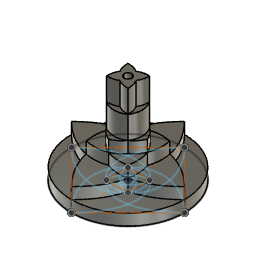
mandala v8 (Autodesk Fusion 360 design; units mm, degrees)
Autodesk Fusion 360 part; units mm, degrees
sketch "Sketch1" plane through (0, 0, 0) normal (0, 0, 1) x (1, 0, 0)
  circle A0 centre (0, 0) radius 25
  line L0 (-25, 0) -> (0, 25)
  line L1 (0, 25) -> (25, 0)
  line L2 (25, 0) -> (0, -25)
  line L3 (0, -25) -> (-25, 0)
  spline S0 degree 4 poles (-25, 0) (0, 25) (25, 0) (0, -25) (-25, 0) knots 0 0 0 0 0 1 1 1 1 1
  line L4 (0, 25) -> (0, -25) construction
  spline S1 degree 4 poles (25, 0) (0, 25) (-25, 0) (0, -25) (25, 0) knots 0 0 0 0 0 1 1 1 1 1
  line L5 (25, 0) -> (0, 25)
  line L6 (0, 25) -> (-25, 0)
  line L7 (-25, 0) -> (0, -25)
  line L8 (0, -25) -> (25, 0)
  line L9 (0, 25) -> (-25, 0)
  line L10 (-25, 0) -> (0, -25)
  line L11 (0, -25) -> (25, 0)
  line L12 (25, 0) -> (0, 25)
  spline S2 degree 4 poles (0, 25) (-25, 0) (0, -25) (25, 0) (0, 25) knots 0 0 0 0 0 1 1 1 1 1
  line L13 (0, -25) -> (25, 0)
  line L14 (25, 0) -> (0, 25)
  line L15 (0, 25) -> (-25, 0)
  line L16 (-25, 0) -> (0, -25)
  spline S3 degree 4 poles (0, -25) (25, 0) (0, 25) (-25, 0) (0, -25) knots 0 0 0 0 0 1 1 1 1 1
  line L17 (-4.7761, 4.7761) -> (4.7922, 4.7652)
  line L18 (4.7922, 4.7652) -> (4.7741, -4.7761)
  line L19 (4.7741, -4.7761) -> (-4.7761, -4.7761)
  line L20 (-4.7761, -4.7761) -> (-4.7761, 4.7761)
  spline S4 degree 4 poles (-4.7761, 4.7761) (4.7922, 4.7652) (4.7741, -4.7761) (-4.7761, -4.7761) (-4.7761, 4.7761) knots 0 0 0 0 0 1 1 1 1 1
  line L21 (4.7922, 4.7652) -> (-4.7761, 4.7761)
  line L22 (-4.7761, 4.7761) -> (-4.7761, -4.7761)
  line L23 (-4.7761, -4.7761) -> (4.7741, -4.7761)
  line L24 (4.7741, -4.7761) -> (4.7922, 4.7652)
  spline S5 degree 4 poles (4.7922, 4.7652) (-4.7761, 4.7761) (-4.7761, -4.7761) (4.7741, -4.7761) (4.7922, 4.7652) knots 0 0 0 0 0 1 1 1 1 1
  line L25 (-4.7761, -4.7761) -> (-4.7761, 4.7761)
  line L26 (-4.7761, 4.7761) -> (4.7922, 4.7652)
  line L27 (4.7922, 4.7652) -> (4.7741, -4.7761)
  line L28 (4.7741, -4.7761) -> (-4.7761, -4.7761)
  spline S6 degree 4 poles (-4.7761, -4.7761) (-4.7761, 4.7761) (4.7922, 4.7652) (4.7741, -4.7761) (-4.7761, -4.7761) knots 0 0 0 0 0 1 1 1 1 1
  line L29 (4.7741, -4.7761) -> (4.7922, 4.7652)
  line L30 (4.7922, 4.7652) -> (-4.7761, 4.7761)
  line L31 (-4.7761, 4.7761) -> (-4.7761, -4.7761)
  line L32 (-4.7761, -4.7761) -> (4.7741, -4.7761)
  spline S7 degree 4 poles (4.7741, -4.7761) (4.7922, 4.7652) (-4.7761, 4.7761) (-4.7761, -4.7761) (4.7741, -4.7761) knots 0 0 0 0 0 1 1 1 1 1
  dimension "d1" = 50
  constraint coincident A0.centre origin
  constraint coincident A0 L0.start
  constraint coincident A0 L0.end
  constraint coincident A0 L1.end
  constraint coincident A0 L2.end
  constraint coincident L0.start L3.end
  constraint coincident L0.end L1.start
  constraint coincident L2.end L3.start
  constraint vertical L4
  constraint symmetric L0.start L4 L1.end
  constraint symmetric S0 L4 S1
  constraint coincident L1.end L2.start
  constraint coincident S3 L17.start
  constraint coincident S1 L17.start
  constraint coincident S3 L17.end
  constraint coincident S2 L19.end
  constraint coincident S1 L19.end
  constraint horizontal L19
  constraint vertical L20
  constraint coincident L17.start L20.end
  constraint coincident L17.end L18.start
  constraint coincident L19.end L20.start
  constraint coincident L18.end L19.start
  constraint horizontal L28
  constraint vertical L31
  constraint horizontal L32
  measures "d1" diameter of A0
extrude "Extrude1" add sketch "Sketch1" along normal blind 5 contours A0 L1 L5 L12 L14 | L1 S1 L5 L12 S2 L14 | A0 L2 L8 L11 L13 | L2 S1 L8 L11 L13 S3 | A0 L0 L6 L9 L15 | L0 S0 L6 L9 S2 L15 | A0 L3 L7 L10 L16 | L3 S0 L7 L10 L16 S3 makes body 1
extrude "Extrude2" add sketch "Sketch1" along normal blind 10 separate body contours S1 S2 S3 | S0 S1 S2 | S0 S1 S3 | S0 S2 S3 picked at (16.3403, 0.2834) picked at (-0.422, 16.3739) picked at (0.2834, -16.3403) makes body 2
extrude "Extrude3" add sketch "Sketch1" along normal blind 15 separate body contours S0 S1 S2 S3 | S0 S1 S2 S3 | S0 S1 S2 S3 | S0 S1 S2 S3 makes body 3
extrude "Extrude4" add sketch "Sketch1" along normal blind 20 separate body contours S0 S1 S3 | S0 S2 S3 L18 L24 S5 L27 L29 | S0 S1 S2 | S1 S2 S3 picked at (-0.4051, 7.5626) picked at (-0.077, -7.5482) picked at (-7.5626, -0.4051) makes body 4
extrude "Extrude5" add sketch "Sketch1" along normal blind 30 separate body contours S0 S3 L17 L21 L26 L30 | S1 L20 L22 L25 L31 | L20 S4 L22 L25 S6 L31 | L17 S4 L21 S5 L26 L30 | S0 L18 L24 L27 L29 | L18 L24 S5 L27 L29 S7 | S2 L19 L23 L28 L32 | L19 L23 L28 S6 L32 S7 makes body 5
extrude "Extrude6" add sketch "Sketch1" along normal blind 40 separate body contours S4 S5 S6 | S5 S6 S7 | S4 S6 S7 | S0 S4 S5 S7 picked at (-3.0447, 3.2066) picked at (3.1772, -3.0696) picked at (-3.1756, -3.068) makes body 6
extrude "Extrude7" add sketch "Sketch1" along normal blind 40 contours S4 S5 S6 S7 | S4 S5 S6 S7 | S4 S5 S6 S7 | S4 S5 S6 S7 | S4 S6 S7 | S5 S6 S7 | S4 S5 S7 | S4 S5 S6 picked at (0.0758, 2.6555) picked at (-2.717, 0.1362) picked at (2.7248, 0.1331) picked at (0.0013, -2.7683) picked at (1.329, 1.561) picked at (-1.319, 1.5624) picked at (1.474, -1.415) bodies 6 5
